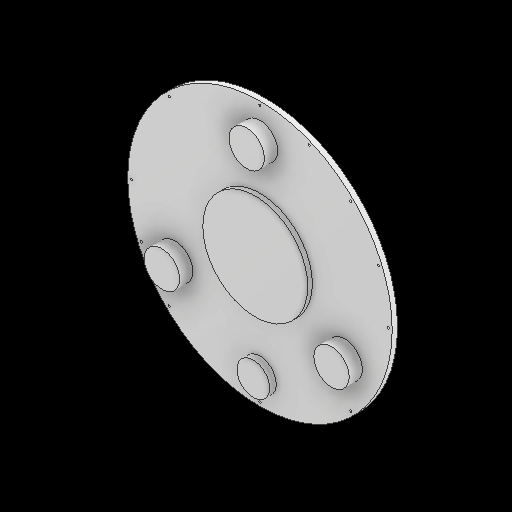
# Autodesk Inventor part: proteox_tube_bottom
Saved by Autodesk Inventor 2026.1 (Build 301233000, 233)
## iProperties
Created: 2025-09-14
Part Number: proteox_tube_bottom
Material: Stainless Steel
Document SubType Name: Modeling
Designer: drago
Density: 8 g/cm^3
Appearance: Smooth - White
Author: drago
Autodesk Inventor part; units mm, degrees
ref_plane "YZ Plane" through (0, 0, 0) normal (1, 0, 0) x (0, 1, 0)
ref_plane "XZ Plane" through (0, 0, 0) normal (0, 1, 0) x (-1, 0, 0)
ref_plane "XY Plane" through (0, 0, 0) normal (0, 0, 1) x (1, 0, 0)
sketch "Sketch7" plane through (0, 0, 0) normal (0, 0, 1) x (1, 0, 0)
  circle A0 centre (0, 0) radius 302.5
  line L0 (0, 0) -> (500, 0) construction
  line L1 (0, 0) -> (433.0127, -250) construction
  line L2 (0, 0) -> (500, 0) construction
  line L3 (0, 0) -> (-433.0127, -250) construction
  line L4 (0, 0) -> (500, 0) construction
  circle A1 centre (0, 224) radius 40.5
  circle A2 centre (-193.9897, -112) radius 40.5
  circle A3 centre (193.9897, -112) radius 40.5
  circle A4 centre (0, -240) radius 37.5
  circle A5 centre (0, 0) radius 120
  circle A6 centre (0, 0) radius 293.8 construction
  line L5 (-461.9398, -191.3417) -> (461.9398, 191.3417) construction
  line L6 (0, 0) -> (191.3417, 461.9398) construction
  line L7 (0, 0) -> (500, 0) construction
  circle A7 centre (0, 293.8) radius 2.5
  circle A8 centre (0, 293.8) radius 4.225 construction
  circle A9 centre (0, 293.8) radius 5 construction
  circle A10 centre (271.4358, 112.4324) radius 5 construction
  circle A11 centre (271.4358, 112.4324) radius 2.5
  line L8 (275.8097, 114.2441) -> (275.1918, 109.5504) construction
  line L9 (275.1918, 109.5504) -> (270.8179, 107.7386) construction
  line L10 (270.8179, 107.7386) -> (267.0619, 110.6207) construction
  line L11 (267.0619, 110.6207) -> (267.6799, 115.3144) construction
  line L12 (267.6799, 115.3144) -> (272.0538, 117.1262) construction
  line L13 (272.0538, 117.1262) -> (275.8097, 114.2441) construction
  circle A12 centre (112.4324, 271.4358) radius 5 construction
  circle A13 centre (112.4324, 271.4358) radius 2.5
  line L14 (114.2441, 275.8097) -> (117.1262, 272.0538) construction
  line L15 (117.1262, 272.0538) -> (115.3144, 267.6799) construction
  line L16 (115.3144, 267.6799) -> (110.6207, 267.0619) construction
  line L17 (110.6207, 267.0619) -> (107.7386, 270.8179) construction
  line L18 (107.7386, 270.8179) -> (109.5504, 275.1918) construction
  line L19 (109.5504, 275.1918) -> (114.2441, 275.8097) construction
  circle A14 centre (-271.4358, -112.4324) radius 5 construction
  circle A15 centre (-271.4358, -112.4324) radius 2.5
  line L20 (-275.8097, -114.2441) -> (-275.1918, -109.5504) construction
  line L21 (-275.1918, -109.5504) -> (-270.8179, -107.7386) construction
  line L22 (-270.8179, -107.7386) -> (-267.0619, -110.6207) construction
  line L23 (-267.0619, -110.6207) -> (-267.6799, -115.3144) construction
  line L24 (-267.6799, -115.3144) -> (-272.0538, -117.1262) construction
  line L25 (-272.0538, -117.1262) -> (-275.8097, -114.2441) construction
  circle A16 centre (-207.748, 207.748) radius 2.5
  circle A17 centre (-207.748, 207.748) radius 4.225 construction
  circle A18 centre (-207.748, 207.748) radius 5 construction
  circle A19 centre (-293.8, 0) radius 2.5
  circle A20 centre (-293.8, 0) radius 4.225 construction
  circle A21 centre (-293.8, 0) radius 5 construction
  circle A22 centre (-207.748, -207.748) radius 2.5
  circle A23 centre (-207.748, -207.748) radius 4.225 construction
  circle A24 centre (-207.748, -207.748) radius 5 construction
  circle A25 centre (0, -293.8) radius 2.5
  circle A26 centre (0, -293.8) radius 4.225 construction
  circle A27 centre (0, -293.8) radius 5 construction
  circle A28 centre (207.748, -207.748) radius 2.5
  circle A29 centre (207.748, -207.748) radius 4.225 construction
  circle A30 centre (207.748, -207.748) radius 5 construction
  circle A31 centre (293.8, 0) radius 2.5
  circle A32 centre (293.8, 0) radius 4.225 construction
  circle A33 centre (293.8, 0) radius 5 construction
  circle A34 centre (207.748, 207.748) radius 2.5
  circle A35 centre (207.748, 207.748) radius 4.225 construction
  circle A36 centre (207.748, 207.748) radius 5 construction
  dimension "d26" = 605
  dimension "d29" = 500
  dimension "d30" = 30
  dimension "d31" = 500
  dimension "d32" = 150
  dimension "d34" = 81
  dimension "d35" = 224
  dimension "d38" = 360
  dimension "d40" = 75
  dimension "d41" = 240
  dimension "d42" = 240
  dimension "d79" = 587.6
  dimension "d80" = 1000
  dimension "d82" = 500
  dimension "d83" = 67.5
  dimension "d84" = 5
  dimension "d85" = 8.45
  dimension "d86" = 10
  dimension "d87" = 10
  dimension "d88" = 5
  dimension "d89" = 8.2
  dimension "d90" = 10
  dimension "d91" = 5
  dimension "d92" = 8.2
  dimension "d93" = 10
  dimension "d94" = 5
  dimension "d95" = 8.2
  dimension "d98" = 360
  constraints: 52 end point, 37 centre point, 25 coincident, 6 point on line, 4 horizontal, 4 point on circle, 3 equal length, 1 midpoint, 95 other
  measures "d26" diameter of A0
  measures "d29" distance of L0.start L1.end
  measures "d30" angle of L1 L2
  measures "d31" distance of L0.start L3.end
  measures "d32" angle of L3 L4
  measures "d34" diameter of A1
  measures "d35" distance of point (0, 0) A1.centre
  measures "d40" diameter of A4
  measures "d41" distance of A4.centre point (0, 0)
  measures "d42" diameter of A5
  measures "d79" diameter of A6
  measures "d80" distance of L5.start L5.end
  measures "d82" distance of L6.start L6.end
  measures "d83" angle of L7 L6
  measures "d84" diameter of A7
  measures "d85" diameter of A8
  measures "d86" diameter of A9
  measures "d87" diameter of A10
  measures "d88" diameter of A11
  measures "d89" distance between parallel lines of L9 L12
  measures "d90" diameter of A12
  measures "d91" diameter of A13
  measures "d92" distance between parallel lines of L15 L18
  measures "d93" diameter of A14
  measures "d94" diameter of A15
  measures "d95" distance between parallel lines of L24 L21
extrude "Extrusion7" add sketch "Sketch7" against normal blind 12.2 contours A0 | A1 | A2 | A3 | A4 | A5 | A7 | A11 | A13 | A15 | A16 | A19 | A22 | A25 | A28 | A31 | A34
extrude "Extrusion8" add sketch "Sketch7" along normal blind 30.25 contours A1 | A2 | A3
extrude "Extrusion9" add sketch "Sketch7" along normal blind 10.7 contours A5
extrude "Extrusion10" add sketch "Sketch7" along normal blind 15.25 contours A4
extrude "Extrusion11" cut sketch "Sketch7" against normal blind 12.2 contours A7 | A11 | A13 | A15 | A16 | A19 | A22 | A25 | A28 | A31 | A34
body "Solid2"
